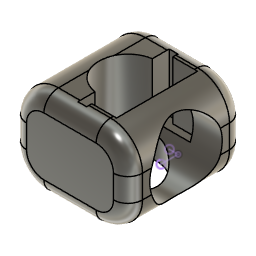
GCPW fixture in plane rotation (Autodesk Fusion 360 design; units mm, degrees)
Autodesk Fusion 360 part; units mm, degrees
sketch "Sketch1" plane through (0, 0, 0) normal (0, 0, 1) x (1, 0, 0)
  line L0 (20, -20) -> (-20, -20)
  line L1 (-20, -20) -> (-20, 20)
  line L2 (-20, 20) -> (20, 20)
  line L3 (20, 20) -> (20, -20)
  line L4 (20, -20) -> (-20, 20) construction
  line L5 (-20, -20) -> (20, 20) construction
  dimension "d1" = 40
  dimension "d2" = 40
  constraint horizontal L0
  constraint perpendicular L0 L1
  constraint parallel L0 L2
  constraint parallel L1 L3
  constraint coincident L4 origin
  constraint coincident L5 origin
  measures "d1" distance of L1.end L2.end
  measures "d2" distance of L0.end L1.end
extrude "Extrude1" add sketch "Sketch1" along normal blind 30
sketch "Sketch2" plane through (0, 0, 30) normal (0, 0, 1) x (-1, 0, 0)
  line L0 (-20, -20) -> (20, -20)
  line L1 (20, -20) -> (20, 20)
  line L2 (20, 20) -> (-20, 20)
  line L3 (-20, 20) -> (-20, -20)
  circle A0 centre (0, 0) radius 7.5
  dimension "d5" = 15
  constraint coincident A0.centre origin
  measures "d5" diameter of A0
extrude "Extrude2" cut sketch "Sketch2" against normal blind 50 contours A0
sketch "Sketch3" plane through (0, 0, 0) normal (0, 0, 1) x (1, 0, 0)
  circle A0 centre (0, 0) radius 10
  dimension "d8" = 20
  constraint coincident A0.centre origin
  measures "d8" diameter of A0
extrude "Extrude3" cut sketch "Sketch3" along normal blind 44
sketch "Sketch4" plane through (0, 0, 0) normal (0, 0, 1) x (1, 0, 0)
ref_plane "WorkPlane1" through (0, 0, 5) normal (0, 0, 1) x (1, 0, 0)
sketch "Sketch5" plane through (0, 0, 5) normal (0, 0, 1) x (1, 0, 0)
  line L0 (1.5, 15.75) -> (-1.5, 15.75)
  line L1 (-1.5, 15.75) -> (-1.5, -15.75)
  line L2 (-1.5, -15.75) -> (1.5, -15.75)
  line L3 (1.5, -15.75) -> (1.5, 15.75)
  line L4 (1.5, 15.75) -> (-1.5, -15.75) construction
  line L5 (-1.5, 15.75) -> (1.5, -15.75) construction
  dimension "d12" = 3
  dimension "d13" = 31.5
  constraint horizontal L0
  constraint perpendicular L0 L1
  constraint parallel L0 L2
  constraint parallel L1 L3
  constraint coincident L4 origin
  constraint coincident L5 origin
  measures "d12" distance of L1.end L2.end
  measures "d13" distance of L0.end L1.end
extrude "Extrude4" cut sketch "Sketch5" along normal blind 40
sketch "Sketch6" plane through (0, 0, 0) normal (0, 0, 1) x (1, 0, 0)
  line L0 (-1.5, 15.75) -> (1.5, 15.75)
  line L1 (1.5, 15.75) -> (1.5, 9.8869)
ref_plane "WorkPlane2" through (0, -12.8184, 5) normal (0, 0, 1) x (1, 0, 0)
sketch "Sketch7" plane through (0, 0, 5) normal (0, 0, 1) x (1, 0, 0)
  line L0 (1.5339, 13.9572) -> (10, 13.9572)
  line L1 (10, 13.9572) -> (10, -14)
  line L2 (10, -14) -> (1.5339, -14)
  line L3 (1.5339, -14) -> (1.5339, 13.9572)
  constraint horizontal L0
  constraint vertical L1
  constraint horizontal L2
  constraint vertical L3
extrude "Extrude5" cut sketch "Sketch7" along normal blind 30
extrude "Extrude6" cut 1 faces at (1.5339, 12.5987, 21.6667) along direction (-1, 0, 0) blind 1
extrude "Extrude7" cut 1 faces at (1.5339, -12.6272, 13.3333) along direction (-1, 0, 0) blind 1
sketch "Sketch8" plane through (20, 0, 0) normal (1, 0, 0) x (0, 1, 0)
  line L0 (-20, 0) -> (20, 0)
  line L1 (20, 0) -> (20, 30)
  line L2 (20, 30) -> (-20, 30)
  line L3 (-20, 30) -> (-20, 0)
  circle A0 centre (0, 15) radius 12.5
  dimension "d26" = 25
  measures "d26" diameter of A0
extrude "Extrude8" cut sketch "Sketch8" against normal blind 12 contours A0
extrude "Extrude9" add 1 faces at (5.0956, -12.4184, 5) along direction (0, 0, 1) blind 5
extrude "Extrude10" add 1 faces at (5.0956, 12.3899, 5) along direction (0, 0, 1) blind 5
sketch "Sketch9" plane through (-20, 0, 0) normal (-1, 0, 0) x (0, -1, 0)
  line L0 (-20, 0) -> (20, 0)
  line L1 (20, 0) -> (20, 30)
  line L2 (20, 30) -> (-20, 30)
  line L3 (-20, 30) -> (-20, 0)
  circle A0 through (12.5, 15, -46) (-6.25, 25.8253, -46) (-6.25, 4.1747, -46)
  dimension "d33" = 25
extrude "Extrude11" cut sketch "Sketch9" along normal blind 27.5 contours A0 in plane through (26, 0, 0) normal (-1, 0, 0)
fillet "Fillet1" radius 11 1 edges at (20, 0, 30)
fillet "Fillet2" radius 11 1 edges at (-20, 0, 30)
fillet "Fillet3" radius 11 1 edges at (-20, 0, 0)
fillet "Fillet4" radius 11 1 edges at (20, 0, 0)
fillet "Fillet5" radius 5 8 edges at (16.7782, -20, 26.7782) (20, -20, 15) (16.7782, -20, 3.2218) (0, -20, 0) (-16.7782, -20, 3.2218) (-20, -20, 15) (-16.7782, -20, 26.7782) (0, -20, 30)
fillet "Fillet6" radius 5 8 edges at (-20, 20, 15) (-16.7782, 20, 3.2218) (0, 20, 0) (16.7782, 20, 3.2218) (20, 20, 15) (16.7782, 20, 26.7782) (0, 20, 30) (-16.7782, 20, 26.7782)
